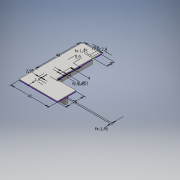
# Autodesk Inventor part: cache_nappe_cote
Saved by Autodesk Inventor 2016 (Build 200138000, 138)
## iProperties
Created: 2018-03-03
Part Number: cache_nappe_cote
Material: Generic
Document SubType Name: Modeling
Designer: Mick
Density: 1 g/cm^3
Appearance: Default
Author: Mick
Autodesk Inventor part; units mm, degrees
ref_plane "YZ Plane" through (0, 0, 0) normal (1, 0, 0) x (0, 1, 0)
ref_plane "XZ Plane" through (0, 0, 0) normal (0, 1, 0) x (-1, 0, 0)
ref_plane "XY Plane" through (0, 0, 0) normal (0, 0, 1) x (1, 0, 0)
sketch "Sketch1" plane through (0, 0, 0) normal (0, 0, 1) x (1, 0, 0)
  line L0 (0, 0) -> (-20, 0)
  line L1 (-20, 0) -> (-20, 48)
  line L2 (-20, 48) -> (0, 48)
  line L3 (0, 48) -> (0, 0)
  line L4 (-20, 0) -> (21, 0)
  line L5 (21, 0) -> (21, -20)
  line L6 (21, -20) -> (-20, -20)
  line L7 (-20, -20) -> (-20, 0)
  line L8 (21, -11.45) -> (-2.55, -11.45)
  line L9 (-2.55, -11.45) -> (-2.55, -8.55)
  line L10 (-2.55, -8.55) -> (21, -8.55)
  line L11 (21, -8.55) -> (21, -11.45)
  line L12 (-2.55, -11.45) -> (-5.45, -11.45)
  line L13 (-5.45, -11.45) -> (-5.45, 41.45)
  line L14 (-5.45, 41.45) -> (-2.55, 41.45)
  line L15 (-2.55, 41.45) -> (-2.55, -11.45)
  line L16 (-2.55, 41.45) -> (-2.55, 38.55)
  line L17 (0, 38.55) -> (0, 41.45)
  line L18 (-12.95, 0) -> (-7.05, 0)
  line L19 (-7.05, 0) -> (-7.05, 25)
  line L20 (-7.05, 25) -> (-12.95, 25)
  line L21 (-12.95, 25) -> (-12.95, 0)
  point P0 (21, -10)
  point P1 (-2.5, 40)
  point P2 (-4, 13.49)
  point P3 (-10, 0)
  point P4 (-10, 48)
  dimension "d0" = 20
  dimension "d1" = 48
  dimension "d2" = 41
  dimension "d3" = 20
  dimension "d5" = 1.45
  dimension "d6" = 2.9
  dimension "d7" = 2.9
  dimension "d8" = 8
  dimension "d11" = 4
  dimension "d12" = 1.45
  dimension "d13" = 1.45
  dimension "d14" = 1.45
  dimension "d16" = 2.95
  dimension "d17" = 5.9
  dimension "d18" = 25
  constraints: 44 end point, 11 parallel, 5 horizontal, 5 perpendicular, 5 point on line, 2 midpoint
  measures "d0" distance of L1.end L2.end
  measures "d1" distance of L0.end L1.end
  measures "d2" distance of L5.end L6.end
  measures "d3" distance of L4.end L5.end
  measures "d5" distance of L8.start point (21, -10)
  measures "d6" distance of L8.end L9.end
  measures "d7" distance of L13.end L14.end
  measures "d8" distance from line of point (-2.5, 40) L2
  measures "d11" distance from line of point (-4, 13.49) L3
  measures "d12" distance from line of L15 point (-4, 13.49)
  measures "d13" distance from line of L13 point (-4, 13.49)
  measures "d14" distance from line of point (-2.5, 40) L14
  measures "d16" distance of L18.start point (-10, 0)
  measures "d17" distance of L20.end L19.end
  measures "d18" distance of L19.end L18.end
extrude "Extrusion1" add sketch "Sketch1" along normal blind 1
extrude "Extrusion2" add sketch "Sketch1" against normal blind 7 contours L13 L14 L15 L0 | L0 L15 L9 L12 L13 | L10 L5 L8 L9
extrude "Extrusion3" add sketch "Sketch1" against normal blind 3 contours L0 L21 L20 L19
equation "\"d5\" = 0.5 * d6"
equation "\"d7\" = d6"
equation "\"d12\" = 0.5 * d6"
equation "\"d14\" = 0.5 * d10"
equation "\"d10\" = d6"
body "Solid1"
